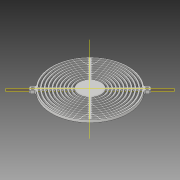
# Autodesk Inventor part: FanGrill
Saved by Autodesk Inventor 2019 (Build 230136000, 136)
## iProperties
Created: 2021-08-20
Part Number: FanGrill
Material: Generic
Document SubType Name: Modeling
Designer: devon
Density: 1 g/cm^3
Appearance: Default
Author: devon
Autodesk Inventor part; units mm, degrees
ref_plane "YZ Plane" through (0, 0, 0) normal (1, 0, 0) x (0, 1, 0)
ref_plane "XZ Plane" through (0, 0, 0) normal (0, 1, 0) x (-1, 0, 0)
sketch "Sketch1" plane through (0, 0, 0) normal (0, 1, 0) x (-1, 0, 0)
  circle A0 centre (0, 0) radius 70
  dimension "d0" = 140
  constraints: 1 centre point, 1 coincident
  measures "d0" diameter of A0
extrude "Extrusion1" add sketch "Sketch1" along normal blind 2.5
ref_plane "Work Plane1" through (0, 0, 0) normal (-0.7071068, 0, 0.7071068) x (0, 1, 0)
sketch "Sketch2" plane through (0, 0, 0) normal (-0.7071068, 0, 0.7071068) x (0, 1, 0)
  line L0 (0, 70) -> (0, -70) projected
  line L1 (2.5, -70) -> (2.5, 70) projected
  line L2 (0, 5) -> (2.5, 5)
  line L3 (2.5, 5) -> (2.5, -5)
  line L4 (2.5, -5) -> (0, -5)
  line L5 (0, -5) -> (0, 5)
  point P0 (0, 0)
  dimension "d5" = 10
  dimension "d6" = 5
  constraints: 8 end point, 2 parallel, 2 point on line, 1 horizontal, 1 perpendicular
  measures "d5" distance between parallel lines of L4 L2
  measures "d6" distance from line of point (0, 0) L4
extrude "Extrusion2" add sketch "Sketch2" along normal mid plane 158
sketch "Sketch4" plane through (0, 0, 0) normal (0, -1, 0) x (1, 0, 0)
  arc A0 (52.9066, -45.8355) -> (-45.8355, 52.9066) centre (0, 0) ccw projected
  line L0 (-59.397, 52.3259) -> (-52.9066, 45.8355) projected
  arc A1 (-45.8355, 52.9066) -> (-52.9066, 45.8355) centre (0, 0) ccw
  line L1 (-52.3259, 59.397) -> (-59.397, 52.3259) projected
  line L2 (-52.9066, 45.8355) -> (-59.397, 52.3259)
  line L3 (-59.397, 52.3259) -> (-52.3259, 59.397)
  line L4 (-52.3259, 59.397) -> (-45.8355, 52.9066)
  line L5 (52.9066, -45.8355) -> (59.397, -52.3259) projected
  arc A2 (45.8355, -52.9066) -> (52.9066, -45.8355) centre (0, 0) ccw
  line L6 (52.9066, -45.8355) -> (59.397, -52.3259)
  line L7 (59.397, -52.3259) -> (52.3259, -59.397) projected
  line L8 (52.3259, -59.397) -> (45.8355, -52.9066)
  constraints: 10 end point, 4 point on circle, 3 perpendicular, 2 centre point, 2 collinear
extrude "Extrusion4" add sketch "Sketch4" along normal blind 2.5
sketch "Sketch5" plane through (0, 2.5, 0) normal (0, 1, 0) x (1, 0, 0)
  circle A0 centre (52.4973, 52.4973) radius 2.625
  circle A1 centre (-52.5027, -52.5027) radius 2.625
  line L0 (-52.3259, -59.397) -> (-59.397, -52.3259) projected
  line L1 (-59.397, -52.3259) -> (-52.9066, -45.8355) projected
  point P0 (0, 0)
  dimension "d19" = 5.25
  dimension "d20" = 5.25
  dimension "d21" = 105
  dimension "d22" = 105
  dimension "d23" = 4.75
  dimension "d24" = 5
  constraints: 2 centre point
  measures "d19" diameter of A1
  measures "d20" diameter of A0
  measures "d21" horizontal distance of A1.centre A0.centre
  measures "d22" horizontal distance of A0.centre A1.centre
  measures "d23" distance from line of L0 A1.centre
  measures "d24" distance from line of L1 A1.centre
extrude "Extrusion5" cut sketch "Sketch5" against normal up to next
sketch "Sketch6" plane through (0, 0, 0) normal (0, -1, 0) x (1, 0, 0)
  circle A0 centre (0, 0) radius 69
  circle A1 centre (0, 0) radius 70
  dimension "d27" = 138
  dimension "d28" = 140
  constraints: 2 centre point, 2 coincident
  measures "d27" diameter of A0
  measures "d28" diameter of A1
extrude "Extrusion6" add sketch "Sketch6" along normal blind 2.5
sketch "Sketch7" plane through (0, 2.5, 0) normal (0, 1, 0) x (1, 0, 0)
  circle A0 centre (0, 0) radius 67.5
  circle A1 centre (0, 0) radius 65
  circle A2 centre (0, 0) radius 62.5
  circle A3 centre (0, 0) radius 60
  circle A4 centre (0, 0) radius 57.5
  circle A5 centre (0, 0) radius 55
  circle A6 centre (0, 0) radius 52.5
  circle A7 centre (0, 0) radius 50
  circle A8 centre (0, 0) radius 47.5
  circle A9 centre (0, 0) radius 45
  circle A10 centre (0, 0) radius 42.5
  circle A11 centre (0, 0) radius 40
  circle A12 centre (0, 0) radius 37.5
  circle A13 centre (0, 0) radius 35
  circle A14 centre (0, 0) radius 32.5
  circle A15 centre (0, 0) radius 30
  circle A16 centre (0, 0) radius 27.5
  circle A17 centre (0, 0) radius 25
  circle A18 centre (0, 0) radius 22.5
  circle A19 centre (0, 0) radius 20
  dimension "d31" = 135
  dimension "d32" = 130
  dimension "d33" = 125
  dimension "d34" = 120
  dimension "d35" = 115
  dimension "d36" = 110
  dimension "d37" = 105
  dimension "d38" = 100
  dimension "d39" = 95
  dimension "d40" = 90
  dimension "d41" = 85
  dimension "d42" = 80
  dimension "d43" = 75
  dimension "d44" = 70
  dimension "d45" = 65
  dimension "d46" = 60
  dimension "d47" = 55
  dimension "d48" = 50
  dimension "d49" = 45
  dimension "d50" = 40
  constraints: 20 centre point, 20 coincident
  measures "d31" diameter of A0
  measures "d32" diameter of A1
  measures "d33" diameter of A2
  measures "d34" diameter of A3
  measures "d35" diameter of A4
  measures "d36" diameter of A5
  measures "d37" diameter of A6
  measures "d38" diameter of A7
  measures "d39" diameter of A8
  measures "d40" diameter of A9
  measures "d41" diameter of A10
  measures "d42" diameter of A11
  measures "d43" diameter of A12
  measures "d44" diameter of A13
  measures "d45" diameter of A14
  measures "d46" diameter of A15
  measures "d47" diameter of A16
  measures "d48" diameter of A17
  measures "d49" diameter of A18
  measures "d50" diameter of A19
extrude "Extrusion7" cut sketch "Sketch7" against normal up to next
ref_plane "Work Plane2" through (0, 0, 0) normal (0.7071068, 0, 0.7071068) x (0, 1, 0)
sketch "Sketch8" plane through (0, 0, 0) normal (-0.7071068, 0, 0.7071068) x (0, 1, 0)
  line L0 (2.5, 57.5) -> (2.5, -57.5) projected
  line L1 (2.5, 2.5) -> (0, 2.5)
  line L2 (0, 2.5) -> (0, -2.5)
  line L3 (0, -2.5) -> (2.5, -2.5)
  line L4 (2.5, -2.5) -> (2.5, 2.5)
  line L5 (3.5, 0) -> (-3.5, 0) projected
  point P0 (0, 0)
  dimension "d54" = 2.5
  dimension "d55" = 5
  constraints: 8 end point, 2 parallel, 1 horizontal, 1 perpendicular, 1 point on line
  measures "d54" distance between parallel lines of L5 L1
  measures "d55" distance between parallel lines of L3 L1
extrude "Extrusion8" add sketch "Sketch8" along normal mid plane 138
sketch "Sketch9" plane through (0, 0, 0) normal (0.7071068, 0, 0.7071068) x (0, 1, 0)
  line L0 (2.5, -19.8431) -> (2.5, 19.8431) projected
  line L1 (0, 19.8431) -> (0, -19.8431) projected
  line L2 (2.5, -2.5) -> (0, -2.5)
  line L3 (0, -2.5) -> (0, 2.5)
  line L4 (0, 2.5) -> (2.5, 2.5)
  line L5 (2.5, 2.5) -> (2.5, -2.5)
  line L6 (-3.5, 0) -> (3.5, 0) projected
  point P0 (0, 0)
  dimension "d58" = 2.5
  dimension "d59" = 5
  constraints: 8 end point, 2 parallel, 2 point on line, 1 horizontal, 1 perpendicular
  measures "d58" distance between parallel lines of L6 L2
  measures "d59" distance between parallel lines of L4 L2
extrude "Extrusion9" add sketch "Sketch9" along normal mid plane 138
fillet "Fillet3" radius 2.375 8 edges at (-52.9066, 0, 45.8355) (-59.397, 0, 52.3259) (-52.3259, 0, 59.397) (-45.8355, 0, 52.9066) (52.9066, 0, -45.8355) (59.397, 0, -52.3259) (52.3259, 0, -59.397) (45.8355, 0, -52.9066)
body "Solid1"
